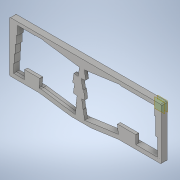
# Autodesk Inventor part: AliceBoardStackedCasePT1
Saved by Autodesk Inventor 2022 (Build 260153000, 153)
## iProperties
Created: 2021-04-11
Part Number: AliceBoardStackedCasePT1
Material: Generic
Document SubType Name: Modeling
Designer: Administrator
Density: 1 g/cm^3
Appearance: Default
Title: Alice Board Case Top v12
Author: Administrator
Autodesk Inventor part; units mm, degrees
ref_plane "YZ Plane" through (0, 0, 0) normal (1, 0, 0) x (0, 1, 0)
ref_plane "XZ Plane" through (0, 0, 0) normal (0, 1, 0) x (-1, 0, 0)
ref_plane "XY Plane" through (0, 0, 0) normal (0, 0, 1) x (1, 0, 0)
ref_plane "Work Plane1" through (323.5667, 111.5783, 0) normal (0, 0, -1) x (-1, 0, 0)
sketch "Sketch1" plane through (323.5667, 111.5783, 0) normal (0, 0, -1) x (-1, 0, 0)
  line L0 (-1, -107.1835) -> (90.6419, -107.1835)
  line L1 (0, -106.1775) -> (90.6419, -106.1775) projected
  line L2 (90.6419, -107.1835) -> (150.3742, -115.5783)
  line L3 (90.6419, -106.1775) -> (150.4165, -114.5783) projected
  line L4 (150.3465, -115.5783) -> (194.8429, -115.5783) projected
  line L5 (150.3742, -115.5783) -> (194.8429, -115.5783)
  line L6 (194.8429, -115.5783) -> (265.5662, -105.6388)
  line L7 (194.7729, -114.5783) -> (265.427, -104.6485) projected
  line L8 (265.5662, -105.6388) -> (327.3907, -105.6388)
  line L9 (327.3907, -105.6388) -> (327.3907, 0)
  line L10 (326.3907, 0) -> (327.3907, 0)
  line L11 (326.3907, 0) -> (-1, 0)
  line L12 (-1, -107.1835) -> (-1, 0)
  line L13 (7.8762, -63.1256) -> (5, -63.1256) projected
  line L14 (5, -101.1775) -> (5, -63.1256)
  line L15 (5, -63.1256) -> (8.8762, -63.1256)
  line L16 (8.8762, -25.0274) -> (10.388, -25.0274) projected
  line L17 (8.8762, -25.0274) -> (11.388, -25.0274)
  line L18 (11.388, -24.0274) -> (11.388, -5.5963) projected
  line L19 (11.388, -5.5963) -> (11.388, -25.0274)
  line L20 (8.8762, -25.0274) -> (8.8762, -63.1256)
  line L21 (5, -101.1775) -> (52.3129, -101.1775) projected
  line L22 (5, -101.1775) -> (52.3129, -101.1775)
  line L23 (52.3129, -101.1775) -> (52.3129, -82.1273) projected
  line L24 (52.3129, -101.1775) -> (52.3129, -82.1273)
  line L25 (90.8058, -100.6856) -> (93.4145, -82.1273) projected
  line L26 (52.3129, -82.1273) -> (93.4145, -82.1273)
  line L27 (165.3463, -111.1977) -> (90.8058, -100.6856) projected
  line L28 (93.4145, -82.1273) -> (90.8058, -100.6856)
  line L29 (90.8058, -100.6856) -> (165.3463, -111.1977)
  line L30 (168.04, -92.097) -> (165.3463, -111.1977) projected
  line L31 (165.3463, -111.1977) -> (168.04, -92.097)
  line L32 (168.9489, -92.2251) -> (168.04, -92.097) projected
  line L33 (168.04, -92.097) -> (168.9489, -92.2251)
  line L34 (171.5736, -73.6138) -> (168.9489, -92.2251) projected
  line L35 (168.9489, -92.2251) -> (171.5736, -73.6138)
  line L36 (164.7689, -72.6541) -> (171.5736, -73.6138) projected
  line L37 (171.5736, -73.6138) -> (164.7689, -72.6541)
  line L38 (164.7689, -72.6541) -> (167.4344, -53.753)
  line L39 (167.9295, -53.8228) -> (165.3338, -72.2289) projected
  line L40 (167.4344, -53.753) -> (169.6975, -54.0722)
  line L41 (167.9295, -53.8228) -> (170.1926, -54.142) projected
  line L42 (169.6975, -54.0722) -> (172.3499, -35.2646) projected
  line L43 (162.9074, -33.9329) -> (172.3499, -35.2646) projected
  line L44 (169.6975, -54.0722) -> (172.3499, -35.2646)
  line L45 (172.3499, -35.2646) -> (162.9074, -33.9329)
  line L46 (162.9074, -33.9329) -> (165.5691, -15.0588)
  line L47 (90.0119, -4.4466) -> (86.5667, -4.4466) projected
  line L48 (165.5691, -15.0588) -> (90.0119, -4.4466)
  line L49 (90.0119, -4.4466) -> (86.5667, -4.4466)
  line L50 (86.5667, -5.5963) -> (86.5667, -4.4466) projected
  line L51 (86.5667, -4.4466) -> (86.5667, -5.5963)
  line L52 (11.388, -5.5963) -> (86.5667, -5.5963) projected
  line L53 (86.5667, -5.5963) -> (11.388, -5.5963)
  line L54 (312.5835, -22.5695) -> (312.5835, -4.072) projected
  line L55 (274.5667, -4.072) -> (274.5667, -3.5004) projected
  line L56 (312.5835, -4.072) -> (274.5667, -4.072)
  line L57 (275.0667, -3.572) -> (274.5667, -4.072) projected
  line L58 (274.5667, -4.072) -> (274.5667, -3.5004)
  line L59 (274.5667, -3.5004) -> (255.4887, -3.5004) projected
  line L60 (274.5667, -3.5004) -> (255.4887, -3.5004)
  line L61 (255.4887, -3.5004) -> (255.4887, -4.4819) projected
  line L62 (255.4887, -3.5004) -> (255.4887, -4.4819)
  line L63 (255.4887, -4.4819) -> (176.5447, -15.5767) projected
  line L64 (255.4887, -4.4819) -> (176.5447, -15.5767)
  line L65 (179.189, -34.3918) -> (188.8101, -33.0397) projected
  line L66 (176.5447, -15.5767) -> (179.189, -34.3918)
  line L67 (188.8101, -33.0397) -> (191.4614, -51.9046) projected
  line L68 (179.189, -34.3918) -> (188.8101, -33.0397)
  line L69 (188.8101, -33.0397) -> (191.4614, -51.9046)
  line L70 (191.4614, -51.9046) -> (187.3114, -52.4878)
  line L71 (189.3979, -70.9266) -> (189.9626, -71.3521) projected
  line L72 (187.3114, -52.4878) -> (189.9626, -71.3521)
  line L73 (181.6626, -72.5186) -> (184.3208, -91.433) projected
  line L74 (189.9626, -71.3521) -> (181.6626, -72.5186)
  line L75 (183.7561, -91.0074) -> (184.3208, -91.433) projected
  line L76 (181.6626, -72.5186) -> (184.3208, -91.433)
  line L77 (184.3208, -91.433) -> (183.1888, -91.5921)
  line L78 (185.8214, -110.3235) -> (261.7781, -99.6485) projected
  line L79 (183.1888, -91.5921) -> (185.8214, -110.3235)
  line L80 (261.813, -100.1485) -> (261.7781, -99.6485) projected
  line L81 (185.8214, -110.3235) -> (261.7781, -99.6485)
  line L82 (266.0502, -100.1485) -> (265.497, -99.6485) projected
  line L83 (261.7781, -99.6485) -> (265.497, -99.6485)
  line L84 (263.5711, -80.6545) -> (297.8916, -80.6545) projected
  line L85 (265.497, -99.6485) -> (263.5711, -80.6545)
  line L86 (263.5711, -80.6545) -> (297.8916, -80.6545)
  line L87 (297.8916, -80.6545) -> (297.8916, -99.6485)
  line L88 (297.8916, -80.6545) -> (297.8916, -99.1545) projected
  line L89 (297.8916, -99.6485) -> (321.3907, -99.6485) projected
  line L90 (297.8916, -99.6485) -> (321.3907, -99.6485)
  line L91 (321.3907, -99.5783) -> (321.3907, -80.6536) projected
  line L92 (321.3907, -99.6485) -> (321.3907, -80.6536)
  line L93 (321.3907, -80.6536) -> (320.0476, -80.6543)
  line L94 (320.0378, -79.6536) -> (320.0378, -61.604) projected
  line L95 (320.0378, -61.604) -> (320.0476, -80.6543)
  line L96 (320.0378, -61.604) -> (318.1009, -61.604)
  line L97 (318.1009, -42.5533) -> (316.2279, -42.5533) projected
  line L98 (318.1009, -42.5533) -> (318.1009, -61.604)
  line L99 (318.1009, -42.5533) -> (315.2279, -42.5533)
  line L100 (315.2279, -23.5695) -> (313.5835, -23.5695) projected
  line L101 (315.2279, -23.5695) -> (315.2279, -42.5533)
  line L102 (312.5835, -4.072) -> (274.5667, -4.072) projected
  line L103 (312.5835, -4.072) -> (312.5835, -23.5695)
  line L104 (315.2279, -23.5695) -> (312.5835, -23.5695)
  line L105 (185.3958, -110.8883) -> (185.8214, -110.3235) projected
  line L106 (165.3463, -111.1977) -> (185.8214, -111.1977)
  line L107 (185.8214, -111.1977) -> (185.8214, -110.3235)
  line L108 (162.9074, -33.9329) -> (165.5691, -15.0588) projected
  line L109 (165.5691, -15.0588) -> (176.5447, -15.0588)
  line L110 (175.98, -15.1512) -> (254.9887, -4.0472) projected
  line L111 (175.98, -15.1512) -> (176.5447, -15.5767) projected
  line L112 (176.5447, -15.5767) -> (176.5447, -15.0588)
  line L113 (330.3907, -105.6388) -> (330.3907, -108.6388)
  line L114 (330.3907, -108.6388) -> (327.3907, -108.6388)
  line L115 (265.5662, -105.6388) -> (265.5662, -108.6388)
  line L116 (327.3907, -108.6388) -> (265.5662, -108.6388)
  line L117 (194.8429, -115.5783) -> (194.8429, -118.5783)
  line L118 (194.8429, -118.5783) -> (265.5662, -108.6388)
  line L119 (150.3465, -115.5783) -> (150.3465, -118.5783)
  line L120 (150.3465, -118.5783) -> (194.8429, -118.5783)
  line L121 (90.6419, -107.1835) -> (90.6395, -110.1835)
  line L122 (150.3465, -118.5783) -> (90.6395, -110.1835)
  line L123 (-4, -107.1835) -> (-4, -110.1835)
  line L124 (-4, -110.1835) -> (-1, -110.1835)
  line L125 (90.6395, -110.1835) -> (-1, -110.1835)
  line L126 (-4, 0) -> (-4, 3)
  line L127 (-4, 3) -> (-1, 3)
  line L128 (-4, 0) -> (-4, -107.1835)
  line L129 (330.3907, 0) -> (330.3907, 3)
  line L130 (330.3907, 3) -> (327.3907, 3)
  line L131 (327.3907, 3) -> (-1, 3)
  line L132 (330.3907, 0) -> (330.3907, -105.6388)
  line L133 (-1, -107.1835) -> (-1, -110.1835)
  line L134 (-1, -107.1835) -> (-4, -107.1835)
  line L135 (327.3907, -105.6388) -> (327.3907, -108.6388)
  line L136 (327.3907, -105.6388) -> (330.3907, -105.6388)
  line L137 (327.3907, 0) -> (327.3907, 3)
  line L138 (327.3907, 0) -> (330.3907, 0)
  line L139 (-1, 0) -> (-1, 3)
  line L140 (-1, 0) -> (-4, 0)
  point P0 (176.5447, -15.0718)
  point P1 (316.2279, -42.5533)
  point P2 (321.3907, -99.5783)
  point P3 (7.8762, -63.1256)
  point P4 (11.388, -24.0274)
  dimension "d1" = 3
  dimension "d2" = 3
  dimension "d3" = 3
  dimension "d4" = 3
  dimension "d5" = 3
  dimension "d7" = 3
  dimension "d8" = 89.954
  dimension "d9" = 3
  dimension "d10" = 3
  dimension "d11" = 3
  dimension "d12" = 3
  dimension "d13" = 3
  dimension "d14" = 3
  dimension "d15" = 331.3907
  constraints: 186 end point, 33 perpendicular, 20 collinear, 7 horizontal, 7 parallel, 3 vertical, 2 point on line
  measures "d1" distance of L113.end L114.end
  measures "d2" distance of L113.start L113.end
  measures "d3" distance of L6.end L115.end
  measures "d4" distance of L4.end L117.end
  measures "d5" distance of L4.start L119.end
  measures "d7" distance of L0.end L121.end
  measures "d8" angle of L0 L121
  measures "d9" distance of L124.end L123.end
  measures "d10" distance of L123.end L123.start
  measures "d11" distance of L126.end L127.end
  measures "d12" distance of L126.start L126.end
  measures "d13" distance of L130.end L129.end
  measures "d14" distance of L129.end L129.start
  measures "d15" distance of L126.end L130.end
extrude "Extrusion1" add sketch "Sketch1" along normal blind 6.35 contours L12 L11 L10 L9 L8 L6 L4 L2 L0 | L134 L128 L140 L12 | L0 L121 L125 L133 | L133 L124 L123 L134 | L2 L4 L119 L122 L121 | L139 L131 L137 L10 L11 | L140 L126 L127 L139 | L4 L117 L120 L119 | L6 L115 L118 L117 | L138 L132 L136 L9 | L137 L130 L129 L138 | L8 L135 L116 L115 | L136 L113 L114 L135 | L30 L32 L34 L36 L38 L40 L42 L43 L46 L109 L112 L110 L111 L66 L65 L67 L70 L72 L74 L73 L77 L79 L107 L106 | L112 L111 L110
ref_plane "Work Plane4" through (323.5667, 111.5783, -6.35) normal (0, 0, -1) x (-1, 0, 0)
fillet "Fillet3" radius 0.5 21 edges at (49, 107.5064, -3.175) (68.0781, 107.0964, -3.175) (10.9833, 88.0088, -3.175) (8.3388, 69.025, -3.175) (5.4658, 49.9744, -3.175) (3.5191, 30.924, -3.175) (133.6041, 40.2262, -3.175) (132.1053, 59.6737, -3.175) (134.7566, 78.5387, -3.175) (139.2459, 20.1453, -3.175) (156.1323, 57.8253, -3.175) (160.6593, 77.6454, -3.175) (158.7979, 38.9242, -3.175) (155.5267, 19.4814, -3.175) (314.6905, 48.4528, -3.175) (312.1788, 86.5509, -3.175) (237, 105.9821, -3.175) (271.2538, 29.451, -3.175) (230.1523, 29.451, -3.175) (59.9956, 30.9238, -3.175) (25.6751, 30.9238, -3.175)
sketch "Sketch3" plane through (323.5667, 111.5783, -6.35) normal (0, 0, -1) x (-1, 0, 0)
  line L0 (-1, -107.1835) -> (90.6419, -107.1835)
  line L1 (90.6419, -107.1835) -> (150.3742, -115.5783)
  line L2 (150.3742, -115.5783) -> (194.8429, -115.5783)
  line L3 (194.8429, -115.5783) -> (265.5662, -105.6388)
  line L4 (265.5662, -105.6388) -> (327.3907, -105.6388)
  line L5 (327.3907, -105.6388) -> (327.3907, 0)
  line L6 (326.3907, 0) -> (327.3907, 0)
  line L7 (326.3907, 0) -> (-1, 0)
  line L8 (-1, -107.1835) -> (-1, 0)
  line L9 (5, -101.1775) -> (5, -63.1256)
  line L10 (5, -63.1256) -> (8.8762, -63.1256)
  line L11 (8.8762, -25.0274) -> (11.388, -25.0274)
  line L12 (11.388, -5.5963) -> (11.388, -25.0274)
  line L13 (8.8762, -25.0274) -> (8.8762, -63.1256)
  line L14 (5, -101.1775) -> (52.3129, -101.1775)
  line L15 (52.3129, -101.1775) -> (52.3129, -82.1273)
  line L16 (52.3129, -82.1273) -> (93.4145, -82.1273)
  line L17 (93.4145, -82.1273) -> (90.8058, -100.6856)
  line L18 (90.8058, -100.6856) -> (165.3463, -111.1977)
  line L19 (165.3463, -111.1977) -> (168.04, -92.097)
  line L20 (168.04, -92.097) -> (168.9489, -92.2251)
  line L21 (168.9489, -92.2251) -> (171.5736, -73.6138)
  line L22 (171.5736, -73.6138) -> (164.7689, -72.6541)
  line L23 (164.7689, -72.6541) -> (167.4344, -53.753)
  line L24 (167.4344, -53.753) -> (169.6975, -54.0722)
  line L25 (169.6975, -54.0722) -> (172.3499, -35.2646)
  line L26 (172.3499, -35.2646) -> (162.9074, -33.9329)
  line L27 (162.9074, -33.9329) -> (165.5691, -15.0588)
  line L28 (165.5691, -15.0588) -> (90.0119, -4.4466)
  line L29 (90.0119, -4.4466) -> (86.5667, -4.4466)
  line L30 (86.5667, -4.4466) -> (86.5667, -5.5963)
  line L31 (86.5667, -5.5963) -> (11.388, -5.5963)
  line L32 (312.5835, -4.0719) -> (274.5667, -4.0719)
  line L33 (274.5667, -4.0719) -> (274.5667, -3.5004)
  line L34 (274.5667, -3.5004) -> (255.4887, -3.5004)
  line L35 (255.4887, -3.5004) -> (255.4887, -4.4819)
  line L36 (255.4887, -4.4819) -> (176.5447, -15.5767)
  line L37 (176.5447, -15.5767) -> (179.189, -34.3918)
  line L38 (179.189, -34.3918) -> (188.8101, -33.0397)
  line L39 (188.8101, -33.0397) -> (191.4614, -51.9046)
  line L40 (191.4614, -51.9046) -> (187.3114, -52.4878)
  line L41 (187.3114, -52.4878) -> (189.9626, -71.3521)
  line L42 (189.9626, -71.3521) -> (181.6626, -72.5186)
  line L43 (181.6626, -72.5186) -> (184.3208, -91.433)
  line L44 (184.3208, -91.433) -> (183.1888, -91.5921)
  line L45 (183.1888, -91.5921) -> (185.8214, -110.3235)
  line L46 (185.8214, -110.3235) -> (261.7781, -99.6485)
  line L47 (261.7781, -99.6485) -> (265.497, -99.6485)
  line L48 (265.497, -99.6485) -> (263.5711, -80.6545)
  line L49 (263.5711, -80.6545) -> (297.8916, -80.6545)
  line L50 (297.8916, -80.6545) -> (297.8916, -99.6485)
  line L51 (297.8916, -99.6485) -> (321.3907, -99.6485)
  line L52 (321.3907, -99.6485) -> (321.3907, -80.6536)
  line L53 (321.3907, -80.6536) -> (320.0476, -80.6543)
  line L54 (320.0378, -61.604) -> (320.0476, -80.6543)
  line L55 (320.0378, -61.604) -> (318.1009, -61.604)
  line L56 (318.1009, -42.5533) -> (318.1009, -61.604)
  line L57 (318.1009, -42.5533) -> (315.2279, -42.5533)
  line L58 (315.2279, -23.5695) -> (315.2279, -42.5533)
  line L59 (312.5835, -4.0719) -> (312.5835, -23.5695)
  line L60 (315.2279, -23.5695) -> (312.5835, -23.5695)
  line L61 (165.3463, -111.1977) -> (185.8214, -111.1977)
  line L62 (185.8214, -111.1977) -> (185.8214, -110.3235)
  line L63 (165.5691, -15.0588) -> (176.5447, -15.0588)
  line L64 (176.5447, -15.5767) -> (176.5447, -15.0588)
  line L65 (330.3907, -105.6388) -> (330.3907, -108.6388)
  line L66 (330.3907, -108.6388) -> (327.3907, -108.6388)
  line L67 (265.5662, -105.6388) -> (265.5662, -108.6388)
  line L68 (327.3907, -108.6388) -> (265.5662, -108.6388)
  line L69 (194.8429, -115.5783) -> (194.8429, -118.5783)
  line L70 (194.8429, -118.5783) -> (265.5662, -108.6388)
  line L71 (150.3465, -115.5783) -> (150.3465, -118.5783)
  line L72 (150.3465, -118.5783) -> (194.8429, -118.5783)
  line L73 (90.6419, -107.1835) -> (90.6395, -110.1835)
  line L74 (150.3465, -118.5783) -> (90.6395, -110.1835)
  line L75 (-4, -107.1835) -> (-4, -110.1835)
  line L76 (-4, -110.1835) -> (-1, -110.1835)
  line L77 (90.6395, -110.1835) -> (-1, -110.1835)
  line L78 (-4, 0) -> (-4, 3)
  line L79 (-4, 3) -> (-1, 3)
  line L80 (-4, 0) -> (-4, -107.1835)
  line L81 (330.3907, 0) -> (330.3907, 3)
  line L82 (330.3907, 3) -> (327.3907, 3)
  line L83 (327.3907, 3) -> (-1, 3)
  line L84 (330.3907, 0) -> (330.3907, -105.6388)
  line L85 (-1, -107.1835) -> (-1, -110.1835)
  line L86 (-1, -107.1835) -> (-4, -107.1835)
  line L87 (327.3907, -105.6388) -> (327.3907, -108.6388)
  line L88 (327.3907, -105.6388) -> (330.3907, -105.6388)
  line L89 (327.3907, 0) -> (327.3907, 3)
  line L90 (327.3907, 0) -> (330.3907, 0)
  line L91 (-1, 0) -> (-1, 3)
  line L92 (-1, 0) -> (-4, 0)
  line L93 (263.6269, -81.2049) -> (265.497, -99.6485) projected
  line L94 (297.8916, -99.6485) -> (297.8916, -81.1545) projected
  line L95 (265.497, -99.6485) -> (297.8916, -99.6485)
  line L96 (52.3129, -101.1775) -> (5, -101.1775) projected
  line L97 (52.3129, -101.1775) -> (90.8069, -101.0676)
  line L98 (90.8058, -100.6856) -> (93.3344, -82.6969) projected
  line L99 (90.8069, -101.0676) -> (90.8058, -100.6856)
  line L100 (330.3907, 3) -> (322.3907, 3)
  line L101 (330.3907, -5) -> (330.3907, 3)
  line L102 (330.3907, -108.6388) -> (323.3907, -108.6388)
  line L103 (323.3907, -108.6388) -> (323.3907, -101.6388)
  line L104 (323.3907, -101.6388) -> (330.3907, -101.6388)
  line L105 (330.3907, -101.6388) -> (330.3907, -108.6388)
  circle A0 centre (323.3907, -101.6388) radius 1.975
  line L106 (330.3907, 3) -> (323.3907, 3)
  line L107 (323.3907, 3) -> (323.3907, -4)
  line L108 (323.3907, -4) -> (330.3907, -4)
  line L109 (330.3907, -4) -> (330.3907, 3)
  circle A1 centre (323.3907, -4) radius 1.975
  line L110 (-4, 3) -> (3, 3)
  line L111 (3, 3) -> (3, -4)
  line L112 (3, -4) -> (-4, -4)
  line L113 (-4, -4) -> (-4, 3)
  line L114 (-4, -110.1835) -> (3, -110.1835)
  line L115 (3, -110.1835) -> (3, -103.1835)
  line L116 (3, -103.1835) -> (-4, -103.1835)
  line L117 (-4, -103.1835) -> (-4, -110.1835)
  circle A2 centre (3, -103.1835) radius 1.975
  circle A3 centre (3, -4) radius 1.975
  dimension "d40" = 3
  dimension "d41" = 3
  dimension "d42" = 3
  dimension "d43" = 3
  dimension "d44" = 3
  dimension "d45" = 3
  dimension "d46" = 89.954
  dimension "d47" = 3
  dimension "d48" = 3
  dimension "d49" = 3
  dimension "d50" = 3
  dimension "d51" = 3
  dimension "d52" = 3
  dimension "d53" = 331.3907
  dimension "d59" = 7
  dimension "d60" = 7
  dimension "d61" = 3.95
  dimension "d62" = 7
  dimension "d63" = 7
  dimension "d64" = 3.95
  dimension "d65" = 7
  dimension "d66" = 7
  dimension "d67" = 7
  dimension "d68" = 7
  dimension "d69" = 3.95
  dimension "d70" = 3.95
  constraints: 228 end point, 34 perpendicular, 12 horizontal, 11 parallel, 4 centre point, 4 coincident, 3 collinear, 3 vertical, 2 point on line
  measures "d40" distance of L65.end L66.end
  measures "d41" distance of L65.start L65.end
  measures "d42" distance of L3.end L67.end
  measures "d43" distance of L2.end L69.end
  measures "d44" distance of L71.start L71.end
  measures "d45" distance of L0.end L73.end
  measures "d46" angle of L0 L73
  measures "d47" distance of L76.end L75.end
  measures "d48" distance of L75.end L75.start
  measures "d49" distance of L78.end L79.end
  measures "d50" distance of L78.start L78.end
  measures "d51" distance of L82.end L81.end
  measures "d52" distance of L81.end L81.start
  measures "d53" distance of L78.end L82.end
  measures "d59" distance of L103.end L104.end
  measures "d60" distance of L102.end L103.end
  measures "d61" diameter of A0
  measures "d62" distance of L108.end L107.end
  measures "d63" distance of L107.end L106.end
  measures "d64" diameter of A1
  measures "d65" distance of L111.end L112.end
  measures "d66" distance of L110.end L111.end
  measures "d67" distance of L116.end L115.end
  measures "d68" distance of L115.end L114.end
  measures "d69" diameter of A2
  measures "d70" diameter of A3
extrude "Extrusion4" add sketch "Sketch3" along normal blind 6.35
fillet "Fillet2" radius 2 4 edges at (327.5667, 1.3948, -6.35) (327.5667, 114.5783, -6.35) (-6.824, 114.5783, -6.35) (-6.824, 2.9395, -6.35)
extrude "Extrusion5" cut sketch "Sketch3" along normal blind 66.675 contours A2 L116 L115 | L115 L116 A2 | A3 L111 L112 | L112 L111 A3 | A1 L108 L107 | L107 L108 A1 | A0 L104 L103 | L103 L104 A0
extrude "Extrusion6" cut sketch "Sketch3" against normal blind 5.8 contours A2 L116 L115 | L115 L116 A2 | A3 L111 L112 | L112 L111 A3 | A1 L108 L107 | L107 L108 A1 | A0 L104 L103 | L103 L104 A0
body "Solid3"
